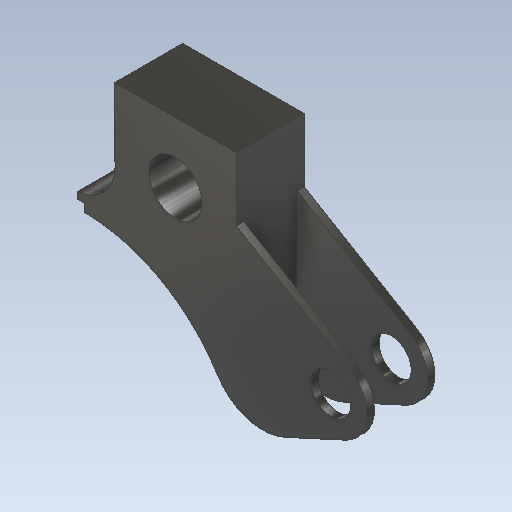
# Autodesk Inventor part: Part28_2
Saved by Autodesk Inventor 2021 (Build 250183000, 183)
## iProperties
Created: 2020-11-13
Part Number: Part28_2
Material: Liga de Nickel-Copper 400
Document SubType Name: Modeling
Designer: Lucas Moura
Density: 8.83 g/cm^3
Appearance: Cromado - Preto polido
Author: Lucas Moura
Autodesk Inventor part; units mm, degrees
ref_plane "YZ Plane" through (0, 0, 0) normal (1, 0, 0) x (0, 1, 0)
ref_plane "XZ Plane" through (0, 0, 0) normal (0, 1, 0) x (-1, 0, 0)
sketch "Sketch1" plane through (0, 0, 0) normal (0, 0, 1) x (1, 0, 0)
  line L0 (0, 0) -> (13.07, 0) construction
  line L1 (13.07, 0) -> (13.07, 20) construction
  line L2 (13.07, 20) -> (0, 20) construction
  line L3 (0, 20) -> (0, 0) construction
  line L4 (0.0102, 11.1339) -> (2.4902, 11.1339) construction
  line L5 (7.0502, 11.1097) -> (11.3067, 8.5922)
  arc A0 (11.1827, 6.1848) -> (11.3067, 8.5922) centre (10.614, 7.421) ccw
  line L6 (2.4702, 13.4954) -> (7.0502, 13.4953)
  line L7 (7.0502, 13.4953) -> (7.0502, 11.1097)
  line L8 (2.4702, 11.0654) -> (2.4702, 13.4954)
  circle A1 centre (4.7602, 11.2054) radius 1
  circle A2 centre (4.7602, 11.2054) radius 2.29 construction
  circle A3 centre (10.614, 7.421) radius 0.75
  line L9 (7.0502, 11.1097) -> (7.0502, 4.2834) construction
  line L10 (11.1827, 6.1848) -> (7.0502, 4.2834)
  arc A4 (1.0511, 9.2211) -> (2.4702, 11.0654) centre (0.8865, 10.8158) ccw
  line L11 (1.0511, 9.2211) -> (1.0511, 8.9911)
  line L12 (1.0511, 8.9911) -> (1.3499, 8.9911)
  line L13 (1.3499, 8.9911) -> (1.3499, 8.6911)
  arc A5 (7.0502, 4.2834) -> (1.3499, 8.6911) centre (1.2762, 2.706) ccw
  point P0 (0, 8.9921)
  point P1 (0, 7.8144)
  point P2 (0, 7.3623)
  dimension "d0" = 20
  dimension "d1" = 13.07
  dimension "d7" = 2
  dimension "d8" = 4.58
  dimension "d11" = 1.5
  dimension "d34" = 0.23
  dimension "d35" = 0.3
  constraints: 28 end point, 6 centre point, 6 point on circle, 6 tangent, 4 vertical, 3 point on line, 2 coincident, 2 horizontal, 2 parallel, 2 perpendicular
  measures "d0" distance of L0.end L1.end
  measures "d1" distance of L1.end L2.end
  measures "d7" diameter of A1
  measures "d8" diameter of A2
  measures "d11" diameter of A3
  measures "d34" distance of L11.start L11.end
  measures "d35" distance of L12.end L13.end
extrude "Extrusion2" add sketch "Sketch1" along normal blind 2.56
ref_plane "Work Plane3" through (11.9729, 7.351, 2.56) normal (0.9986772, -0.0514186, 0) x (0.0514186, 0.9986772, 0)
sketch "Sketch5" plane through (11.9729, 7.351, 2.56) normal (0.9986772, -0.0514186, 0) x (0.0514186, 0.9986772, 0)
  line L0 (3.5006, -2.56) -> (3.5006, 0) projected
  line L1 (3.5006, -1.28) -> (3.5006, -0.28)
  line L2 (3.5006, -0.28) -> (3.5006, -1.28)
  line L3 (3.5006, -1.28) -> (3.5006, -2.28)
  line L4 (3.5006, -0.28) -> (-3.2437, -0.28)
  line L5 (-3.2437, -0.28) -> (-3.2437, -2.28)
  line L6 (3.5006, -2.28) -> (-3.2437, -2.28)
  point P0 (-7.9569, -2.56)
  dimension "d29" = 1
  dimension "d30" = 1
  constraints: 12 end point, 2 point on line, 1 collinear, 1 midpoint, 1 perpendicular
  measures "d29" distance of L1.start L1.end
  measures "d30" distance of L1.start L3.end
extrude "Extrusion6" cut sketch "Sketch5" against normal up to surface surface through (7.0502, 11.1097, 0) normal (1, -0.000029, 0)
fillet "Fillet3" radius 2 1 edges at (7.0502, 4.2834, 1.28)
body "Solid2"
